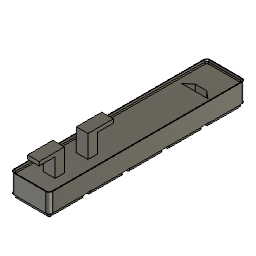
charging_brick_tie_5x1 (Autodesk Fusion 360 design; units mm, degrees)
part number: 2026-05-09-16-48-30-027
Autodesk Fusion 360 part; units mm, degrees
ref_plane "WorkPlane1" through (0, 0, 0) normal (0, 0, 1) x (1, 0, 0)
sketch "Base plate sketch" plane through (0, 0, 0) normal (0, 0, 1) x (1, 0, 0)
  line L0 (-0.25, -0.25) -> (41.75, -0.25)
  line L1 (41.75, -0.25) -> (41.75, 41.75)
  line L2 (41.75, 41.75) -> (-0.25, 41.75)
  line L3 (-0.25, 41.75) -> (-0.25, -0.25)
  dimension "d2" = 0.25
  dimension "d3" = 0.25
  dimension "d4" = 42
  dimension "d5" = 42
  constraint horizontal L0
  constraint vertical L1
  constraint horizontal L2
  constraint vertical L3
  measures "d2" vertical distance of origin L0.start
  measures "d3" horizontal distance of origin L2.end
  measures "d4" horizontal distance of L0.start L0.end
  measures "d5" vertical distance of L0.end L1.end
extrude "Base top section extrude" add sketch "Base plate sketch" against normal blind 2.4 makes body 1
fillet "Base corner fillet" radius 4 8 edges at (-0.25, -0.25, -1.2) (41.75, -0.25, -1.2) (41.75, -0.25, -1.2) (41.75, 41.75, -1.2) (41.75, 41.75, -1.2) (-0.25, 41.75, -1.2) (-0.25, 41.75, -1.2) (-0.25, -0.25, -1.2) on bodies 1
chamfer "Chamfer1" distance 2.4 angle 45 8 edges at (0.9216, 40.5784, -2.4) (-0.25, 20.75, -2.4) (0.9216, 0.9216, -2.4) (20.75, -0.25, -2.4) (40.5784, 0.9216, -2.4) (41.75, 20.75, -2.4) (40.5784, 40.5784, -2.4) (20.75, 41.75, -2.4) on bodies 1
extrude "Extrude2" add 1 faces at (15.6168, 15.0833, -2.4) along direction (0, 0, -1) blind 2.6 on bodies 1 bodies 1
chamfer "Chamfer2" distance 0.8 angle 45 8 edges at (2.6186, 38.8814, -5) (20.75, 39.35, -5) (38.8814, 38.8814, -5) (39.35, 20.75, -5) (38.8814, 2.6186, -5) (20.75, 2.15, -5) (2.6186, 2.6186, -5) (2.15, 20.75, -5) on bodies 1
pattern_linear "R-Pattern1" count 1 spacing 42 along (1, 0, 0) count 5 spacing 42 along (0, 1, 0) of bodies 1 makes body 2 at (26.4167, 55.75, 0) makes body 3 at (26.4167, 97.75, 0) makes body 4 at (26.4167, 139.75, 0) makes body 5 at (26.4167, 181.75, 0)
sketch "Simple box sketch" plane through (0, 0, 0) normal (0, 0, 1) x (1, 0, 0)
  line L0 (0, 0) -> (41.5, 0)
  line L1 (41.5, 0) -> (41.5, 209.5)
  line L2 (41.5, 209.5) -> (0, 209.5)
  line L3 (0, 209.5) -> (0, 0)
  dimension "d18" = 41.5
  dimension "d19" = 209.5
  constraint horizontal L0
  constraint vertical L1
  constraint horizontal L2
  constraint vertical L3
  constraint coincident L0.start L3
  constraint coincident L3.end L0
  measures "d18" horizontal distance of L0.start L0.end
  measures "d19" vertical distance of L0.end L1.end
extrude "Simple box extrude" add sketch "Simple box sketch" along normal blind 16 separate body makes body 6
fillet "Bin body corner fillets" radius 3.75 8 edges at (0, 0, 8) (0, 209.5, 8) (41.5, 209.5, 8) (41.5, 0, 8) (41.5, 0, 8) (0, 0, 8) (0, 209.5, 8) (41.5, 209.5, 8) on bodies 6
ref_plane "WorkPlane2" through (0, 0, 16) normal (0, 0, 1) x (1, 0, 0)
sketch "Simple box at point sketch" plane through (0, 0, 16) normal (0, 0, 1) x (1, 0, 0)
  line L0 (0, 0) -> (41.5, 0)
  line L1 (41.5, 0) -> (41.5, 209.5)
  line L2 (41.5, 209.5) -> (0, 209.5)
  line L3 (0, 209.5) -> (0, 0)
  dimension "d25" = 41.5
  dimension "d26" = 209.5
  constraint horizontal L0
  constraint vertical L1
  constraint horizontal L2
  constraint vertical L3
  constraint coincident L0.start L3
  constraint coincident L3.end L0
  measures "d25" horizontal distance of L0.start L0.end
  measures "d26" vertical distance of L0.end L1.end
extrude "Simple box at point extrude" add sketch "Simple box at point sketch" along normal blind 4.4 separate body makes body 7
fillet "Lip body corner fillets" radius 3.75 8 edges at (41.5, 0, 18.2) (0, 0, 18.2) (0, 209.5, 18.2) (41.5, 209.5, 18.2) (41.5, 209.5, 18.2) (41.5, 0, 18.2) (0, 0, 18.2) (0, 209.5, 18.2) on bodies 7
ref_plane "WorkPlane3" through (0, 0, 21) normal (0, 0, 1) x (1, 0, 0)
sketch "Base plate sketch (1)" plane through (0, 0, 21) normal (0, 0, 1) x (1, 0, 0)
  line L0 (-0.5, -0.5) -> (42, -0.5)
  line L1 (42, -0.5) -> (42, 210)
  line L2 (42, 210) -> (-0.5, 210)
  line L3 (-0.5, 210) -> (-0.5, -0.5)
  dimension "d32" = 0.5
  dimension "d33" = 0.5
  dimension "d34" = 42.5
  dimension "d35" = 210.5
  constraint horizontal L0
  constraint vertical L1
  constraint horizontal L2
  constraint vertical L3
  measures "d32" vertical distance of origin L0.start
  measures "d33" horizontal distance of origin L2.end
  measures "d34" horizontal distance of L0.start L0.end
  measures "d35" vertical distance of L0.end L1.end
extrude "Base top section extrude (1)" add sketch "Base plate sketch (1)" against normal blind 2.4 separate body makes body 8
fillet "Base corner fillet (1)" radius 4.25 8 edges at (-0.5, -0.5, 19.8) (42, -0.5, 19.8) (42, -0.5, 19.8) (42, 210, 19.8) (42, 210, 19.8) (-0.5, 210, 19.8) (-0.5, 210, 19.8) (-0.5, -0.5, 19.8) on bodies 8
chamfer "Chamfer3" distance 2.4 angle 45 8 edges at (0.7448, 208.7552, 18.6) (-0.5, 104.75, 18.6) (0.7448, 0.7448, 18.6) (20.75, -0.5, 18.6) (40.7552, 0.7448, 18.6) (42, 104.75, 18.6) (40.7552, 208.7552, 18.6) (20.75, 210, 18.6) on bodies 8
extrude "Extrude6" add 1 faces at (27.0335, 71.0833, 18.6) along direction (0, 0, -1) blind 2.6 on bodies 8 bodies 8
ref_plane "WorkPlane4" through (20.75, 104.75, 20.4) normal (0, 0, 1) x (1, 0, 0)
sketch "Lip top chamfer" plane through (0, 0, 20.4) normal (0, 0, 1) x (1, 0, 0)
  line L0 (0, 0) -> (41.5, 0)
  line L1 (41.5, 0) -> (41.5, 209.5)
  line L2 (41.5, 209.5) -> (0, 209.5)
  line L3 (0, 209.5) -> (0, 0)
  dimension "d44" = 41.5
  dimension "d45" = 209.5
  constraint horizontal L0
  constraint vertical L1
  constraint horizontal L2
  constraint vertical L3
  constraint coincident L0.start L3
  constraint coincident L3.end L0
  measures "d44" horizontal distance of L0.start L0.end
  measures "d45" vertical distance of L0.end L1.end
extrude "Lip top chamfer cut" add sketch "Lip top chamfer" against normal blind 0.6 separate body makes body 9
combine "Combine1" operation cut target body 7 tool bodies 9 8
ref_plane "WorkPlane5" through (0, 0, 16) normal (0, 0, 1) x (1, 0, 0)
sketch "Simple box at point sketch (1)" plane through (0, 0, 16) normal (0, 0, 1) x (1, 0, 0)
  line L0 (1.2, 1.2) -> (40.3, 1.2)
  line L1 (40.3, 1.2) -> (40.3, 208.3)
  line L2 (40.3, 208.3) -> (1.2, 208.3)
  line L3 (1.2, 208.3) -> (1.2, 1.2)
  dimension "d49" = 1.2
  dimension "d50" = 1.2
  dimension "d51" = 39.1
  dimension "d52" = 207.1
  constraint horizontal L0
  constraint vertical L1
  constraint horizontal L2
  constraint vertical L3
  measures "d49" vertical distance of origin L0.start
  measures "d50" horizontal distance of origin L2.end
  measures "d51" horizontal distance of L0.start L0.end
  measures "d52" vertical distance of L0.end L1.end
extrude "Lip bottom chamfer extrude" add sketch "Simple box at point sketch (1)" along normal blind 2.55 separate body makes body 10
fillet "Fillet5" radius 2.55 8 edges at (1.2, 1.2, 17.275) (1.2, 208.3, 17.275) (1.2, 208.3, 17.275) (40.3, 208.3, 17.275) (40.3, 1.2, 17.275) (1.2, 1.2, 17.275) (40.3, 208.3, 17.275) (40.3, 1.2, 17.275) on bodies 10
chamfer "Chamfer4" distance 2.55 angle 45 8 edges at (1.9469, 1.9469, 18.55) (20.75, 1.2, 18.55) (39.5531, 1.9469, 18.55) (40.3, 104.75, 18.55) (39.5531, 207.5531, 18.55) (20.75, 208.3, 18.55) (1.9469, 207.5531, 18.55) (1.2, 104.75, 18.55) on bodies 10
combine "Combine2" operation cut target body 7 tool bodies 10
combine "Combine3" operation add target body 6 tool bodies 7
ref_plane "WorkPlane6" through (0, 0, 0) normal (0, 0, 1) x (1, 0, 0)
sketch "Base clearance cut sketch" plane through (0, 0, 0) normal (0, 0, 1) x (1, 0, 0)
  line L0 (3.75, 0) -> (37.75, 0)
  line L1 (41.5, 3.75) -> (41.5, 205.75)
  line L2 (37.75, 209.5) -> (3.75, 209.5)
  line L3 (0, 205.75) -> (0, 3.75)
  arc A0 (37.75, 0) -> (41.5, 3.75) centre (37.75, 3.75) ccw
  arc A1 (41.5, 205.75) -> (37.75, 209.5) centre (37.75, 205.75) ccw
  arc A2 (3.75, 209.5) -> (0, 205.75) centre (3.75, 205.75) ccw
  arc A3 (0, 3.75) -> (3.75, 0) centre (3.75, 3.75) ccw
  arc A4 (37.75, -10) -> (51.5, 3.75) centre (37.75, 3.75) ccw
  line L4 (51.5, 3.75) -> (51.5, 205.75)
  arc A5 (51.5, 205.75) -> (37.75, 219.5) centre (37.75, 205.75) ccw
  line L5 (37.75, 219.5) -> (3.75, 219.5)
  arc A6 (3.75, 219.5) -> (-10, 205.75) centre (3.75, 205.75) ccw
  line L6 (-10, 205.75) -> (-10, 3.75)
  arc A7 (-10, 3.75) -> (3.75, -10) centre (3.75, 3.75) ccw
  line L7 (3.75, -10) -> (37.75, -10)
  point P0 (41.5, 0)
  point P1 (41.5, 209.5)
  dimension "d59" = 41.5
  dimension "d60" = 209.5
  dimension "d61" = 3.75
  dimension "d62" = 10
  constraint horizontal L0
  constraint vertical L1
  constraint horizontal L2
  constraint vertical L3
  constraint coincident origin L3
  constraint coincident origin L0
  constraint coincident P0 L0
  constraint coincident P0 L1
  constraint tangent L0 A0
  constraint tangent L1 A0
  constraint coincident P1 L1
  constraint coincident P1 L2
  constraint tangent L1 A1
  constraint tangent L2 A1
  constraint tangent L2 A2
  constraint tangent L3 A2
  constraint tangent L3 A3
  constraint tangent L0 A3
  constraint equal A0 A1
  constraint equal A1 A2
  constraint equal A2 A3
  measures "d59" horizontal distance of origin P0
  measures "d60" vertical distance of P0 P1
  measures "d61" radius of A0
extrude "Base side clearance cut" cut sketch "Base clearance cut sketch" along normal blind 1000 and the other way blind 1000 bodies 1 2 3 4 5 6
combine "Combine4" operation add target body 6 tool bodies 2 3 4 5 1 1
ref_plane "WorkPlane7" through (20.75, 104.75, 16) normal (0, 0, 1) x (1, 0, 0)
sketch "Sketch8" plane through (0, 0, 16) normal (0, 0, 1) x (1, 0, 0)
  line L0 (14.6, 182.6) -> (26.8, 182.6)
  line L1 (26.8, 175.9) -> (39.6, 175.9)
  circle A0 centre (39.6, 175.9) radius 4.8
  line L2 (26.8, 182.6) -> (34.8, 175.9)
  line L3 (26.8, 175.9) -> (1.9, 175.9)
  circle A1 centre (1.9, 175.9) radius 4.8
  line L4 (14.6, 182.6) -> (6.7, 175.9)
  dimension "d71" = 12.2
  dimension "d72" = 6.7
  dimension "d73" = 9.6
  dimension "d74" = 9.6
  constraint horizontal L0
  constraint coincident L1.end A0.centre
  constraint coincident A0 L2.end
  constraint coincident L1 L2.end
  constraint coincident L3.end A1.centre
  constraint coincident L3 L4.end
  constraint coincident A1 L4.end
  measures "d71" distance of L0.start L0.end
  measures "d72" distance of L0.end L1.start
  measures "d73" diameter of A0
  measures "d74" diameter of A1
extrude "Extrude10" cut sketch "Sketch8" against normal blind 19 contours L0 L1 L2 L3 L4 bodies 6
sketch "Sketch9" plane through (0, 0, 16) normal (0, 0, 1) x (-1, 0, 0)
  line L0 (-6.7, -175.9) -> (-14.6, -182.6)
  line L1 (-14.6, -182.6) -> (-26.8, -182.6)
  line L2 (-26.8, -182.6) -> (-34.8, -175.9)
  line L3 (-34.8, -175.9) -> (-6.7, -175.9)
  line L4 (-3.75, -1.2) -> (-37.75, -1.2)
  arc A0 (-37.75, -1.2) -> (-40.3, -3.75) centre (-37.75, -3.75) ccw
  line L5 (-40.3, -3.75) -> (-40.3, -205.75)
  arc A1 (-40.3, -205.75) -> (-37.75, -208.3) centre (-37.75, -205.75) ccw
  line L6 (-37.75, -208.3) -> (-3.75, -208.3)
  arc A2 (-3.75, -208.3) -> (-1.2, -205.75) centre (-3.75, -205.75) ccw
  line L7 (-1.2, -205.75) -> (-1.2, -3.75)
  arc A3 (-1.2, -3.75) -> (-3.75, -1.2) centre (-3.75, -3.75) ccw
  line L8 (-34.8, -175.9) -> (-34.8147, -95.9)
  line L9 (-39.6, -95.9) -> (-1.9, -95.875)
  line L10 (-34.8259, -66.0076) -> (-1.8986, -65.9953)
  line L11 (-34.8297, -55.9) -> (-2, -55.9)
  line L12 (-14.5, -55.9) -> (-14.5, -66)
  line L13 (-27, -55.9) -> (-27, -66.0047)
  line L14 (-34.8391, -31) -> (-1.9, -31)
  line L15 (-34.8429, -20.9) -> (-1.9, -20.9)
  line L16 (-26.9, -20.9) -> (-26.9, -31)
  line L17 (-14.4, -20.9) -> (-14.4, -31)
  dimension "d77" = 80
  dimension "d79" = 37.7
  constraint coincident L2.end L3.start
  constraint perpendicular L7 L11
  constraint coincident L11 L12.start
  constraint coincident L10 L12.end
  constraint coincident L11 L13.start
  constraint coincident L10 L13.end
  constraint horizontal L14
  constraint perpendicular L7 L15
  constraint coincident L15 L16.start
  constraint coincident L14 L16.end
  constraint coincident L15 L17.start
  constraint coincident L14 L17.end
  measures "d77" distance of L2.end L8.end
  measures "d79" horizontal distance of L9.start L9.end
extrude "Extrude11" add sketch "Sketch9" along normal blind 20 contours L10 L11 L12 L13 | L14 L15 L16 L17 bodies 6
ref_plane "WorkPlane8" through (20.65, 25.95, 36) normal (0, 0, 1) x (1, 0, 0)
sketch "Sketch10" plane through (0, 0, 36) normal (0, 0, 1) x (1, 0, 0)
  line L0 (26.9, 20.9) -> (26.9, 3.9)
  line L1 (26.9, 3.9) -> (14.4, 3.9)
  line L2 (14.4, 3.9) -> (14.4, 31)
  line L3 (14.4, 31) -> (26.9, 31)
  line L4 (26.9, 31) -> (26.9, 3.9)
  dimension "d91" = 17
  constraint vertical L0
  constraint horizontal L1
  constraint vertical L2
  constraint horizontal L3
  constraint vertical L4
  measures "d91" distance of L0.start L0.end
extrude "Extrude12" add sketch "Sketch10" along normal blind 4 bodies 6
ref_plane "WorkPlane9" through (20.75, 60.9523, 36) normal (0, 0, 1) x (1, 0, 0)
sketch "Sketch11" plane through (0, 0, 36) normal (0, 0, 1) x (1, 0, 0)
  line L0 (27, 66) -> (27, 83)
  line L1 (27, 83) -> (14.5, 83)
  line L2 (14.5, 83) -> (14.5, 55.9)
  line L3 (14.5, 55.9) -> (27, 55.9)
  line L4 (27, 55.9) -> (27, 83)
  constraint vertical L0
  constraint horizontal L1
  constraint vertical L2
  constraint horizontal L3
  constraint vertical L4
extrude "Extrude13" add sketch "Sketch11" along normal blind 4 bodies 6
equation "d6 = -( 2.40 mm )"
equation "d36 = -( 2.40 mm )"
equation "d46 = -( 0.60 mm )"
named bodies: "Base", "Base (1)", "Base (2)", "Base (3)", "Base (4)", "Gridfinity bin 5x1x3", "Lip body", "Lip cutout"
